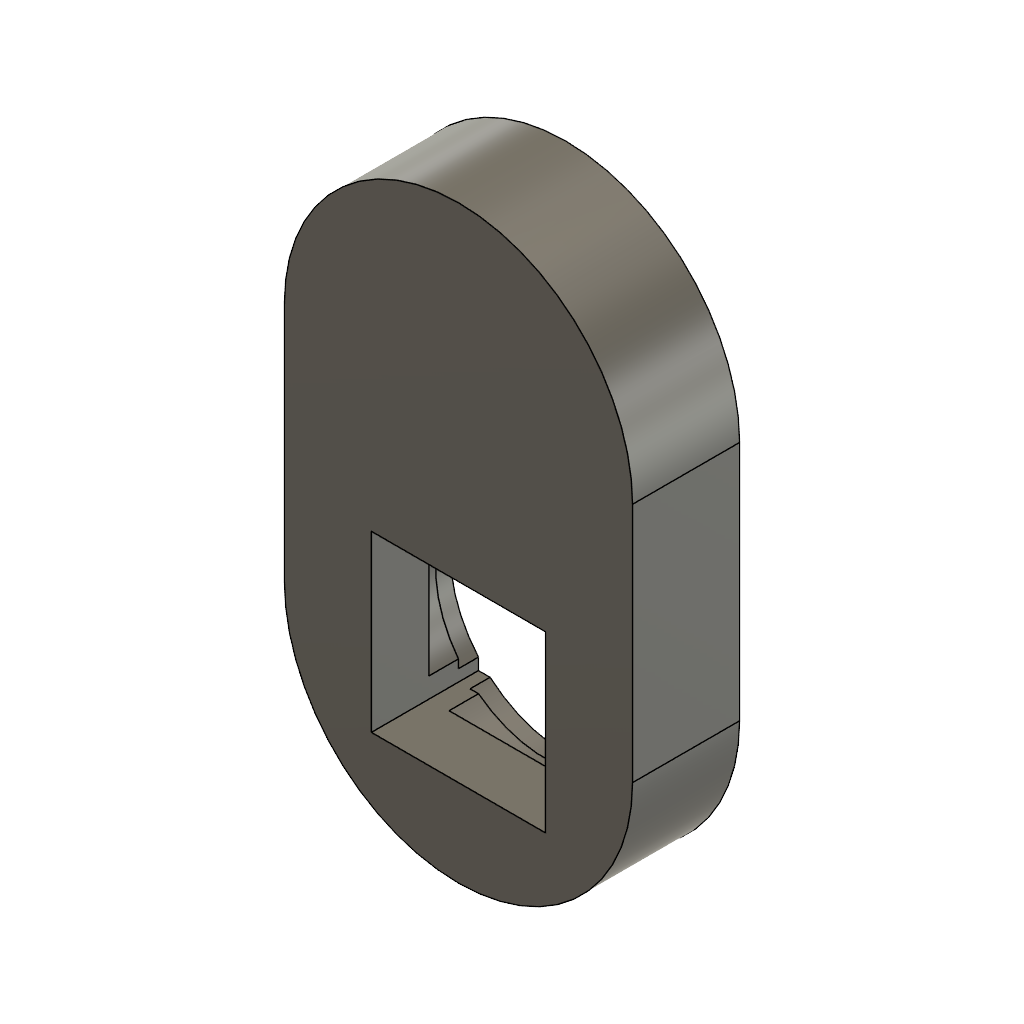
microscopio (Autodesk Fusion 360 design; units mm, degrees)
part number: 2026-09-25-17-02-42-894
Autodesk Fusion 360 part; units mm, degrees
note: some values were not read from the file. Set by a fixed rule: which sketch regions a step uses.
sketch "Boceto1" plane through (0, 0, 0) normal (0, 0, 1) x (1, 0, 0)
  circle A0 centre (0, 9) radius 13
  circle A1 centre (0, -9) radius 13
  line L0 (-13, -9) -> (-13, 9)
  line L1 (13, -9) -> (13, 9)
extrude "Extruir1" add sketch "Boceto1" along normal blind 8
sketch "Boceto2" plane through (0, 0, 0) normal (0, 0, 1) x (1, 0, 0)
  circle A0 centre (0, 9) radius 8.6
  circle A1 centre (0, -9) radius 8.6
  line L0 (-8.6, -9) -> (-8.6, 9)
  line L1 (8.6, -9) -> (8.6, 9)
extrude "Extruir2" cut sketch "Boceto2" along normal blind 1.5
sketch "Boceto3" plane through (0, 0, 0) normal (0, 0, 1) x (1, 0, 0)
  circle A0 centre (0, 9) radius 8.2
  circle A1 centre (0, -9) radius 8.2
extrude "Extruir3" cut sketch "Boceto3" along normal blind 3.7
sketch "Boceto4" plane through (0, 0, 0) normal (0, 0, 1) x (1, 0, 0)
  line L0 (-6.5, -15.5) -> (6.5, -15.5)
  line L1 (6.5, -15.5) -> (6.5, -2.5)
  line L2 (6.5, -2.5) -> (-6.5, -2.5)
  line L3 (-6.5, -2.5) -> (-6.5, -15.5)
extrude "Extruir4" cut sketch "Boceto4" along normal blind 8
